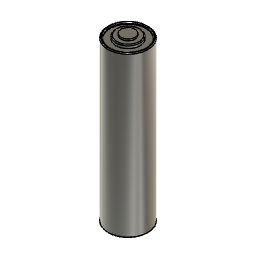
pilha AA v1 (Autodesk Fusion 360 design; units mm, degrees)
Autodesk Fusion 360 part; units mm, degrees
sketch "Sketch1" plane through (0, 0, 0) normal (0, 0, 1) x (1, 0, 0)
  circle A0 centre (0, 0) radius 2.5
  dimension "d1" = 5
  constraint coincident A0.centre origin
  measures "d1" diameter of A0
extrude "Extrude1" add sketch "Sketch1" along normal blind 20
fillet "Fillet1" radius 0.1 1 edges at (-2.3308, -0.904, 0)
fillet "Fillet2" radius 0.1 1 edges at (-2.3308, -0.904, 20)
sketch "Sketch2" plane through (0, 0, 20) normal (0, 0, 1) x (-1, 0, 0)
  circle A0 centre (0, 0) radius 2.4
  circle A1 centre (0, 0) radius 2.25
  dimension "d8" = 4.5
  constraint coincident A0.centre A1.centre
  measures "d8" diameter of A1
extrude "Extrude2" cut sketch "Sketch2" against normal blind 0.2 contours A1
fillet "Fillet3" radius 0.1 1 edges at (2.0977, -0.8136, 20)
sketch "Sketch3" plane through (0, 0, 19.8) normal (0, 0, 1) x (-1, 0, 0)
  circle A0 centre (0, 0) radius 2.25
  circle A1 centre (0, 0) radius 1
  dimension "d13" = 2
  constraint coincident A0.centre A1.centre
  measures "d13" diameter of A1
extrude "Extrude3" add sketch "Sketch3" along normal blind 0.4 contours A1
fillet "Fillet4" radius 0.1 1 edges at (0.9323, 0.3616, 20.2)
move_face "OffsetFaces1" offset 0.5 1 faces at (-0.9988, 0.0498, 19.9)
sketch "Sketch4" plane through (0, 0, 20.2) normal (0, 0, 1) x (-1, 0, 0)
  circle A0 centre (0, 0) radius 1.4
  circle A1 centre (0, 0) radius 0.875
  dimension "d19" = 1.75
  constraint coincident A0.centre A1.centre
  measures "d19" diameter of A1
extrude "Extrude4" add sketch "Sketch4" along normal blind 0.2 contours A1
sketch "Sketch5" plane through (0, 0, 0) normal (0, 0, -1) x (1, 0, 0)
  circle A0 centre (0, 0) radius 2.4
  circle A1 centre (0, 0) radius 1.75
  dimension "d22" = 3.5
  constraint coincident A0.centre A1.centre
  measures "d22" diameter of A1
extrude "Extrude5" cut sketch "Sketch5" against normal blind 0.1
extrude "Extrude6" add 1 faces at (0.9096, -0.438, 0) along direction (0, 0, -1) blind 0.1
fillet "Fillet5" radius 0.1 1 edges at (-1.6316, 0.6328, -0.1)
